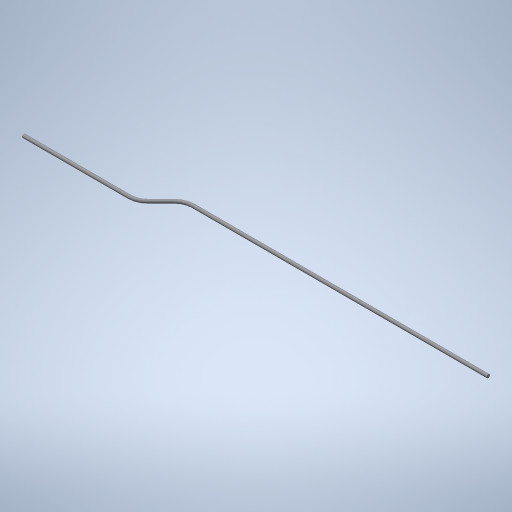
# Autodesk Inventor part: cable medio
Saved by Autodesk Inventor 2023 (Build 270158000, 158)
## iProperties
Created: 2022-10-18
Part Number: cable medio
Material: Generic
Document SubType Name: Modeling
Designer: Xiaba
Density: 1 g/cm^3
Appearance: Default
Author: Xiaba
Autodesk Inventor part; units mm, degrees
ref_plane "YZ Plane" through (0, 0, 0) normal (1, 0, 0) x (0, 1, 0)
ref_plane "XZ Plane" through (0, 0, 0) normal (0, 1, 0) x (-1, 0, 0)
ref_plane "XY Plane" through (0, 0, 0) normal (0, 0, 1) x (1, 0, 0)
sketch "Sketch1" plane through (0, 0, 0) normal (1, 0, 0) x (0, 1, 0)
  circle A0 centre (0, 0) radius 0.45
  dimension "d0" = 0.9
  constraints: 1 centre point, 1 coincident
  measures "d0" diameter of A0
sketch "Sketch2" plane through (0, 0, 0) normal (0, 1, 0) x (-1, 0, 0)
  line L0 (0, 0) -> (0.1, 0)
  line L1 (0.1, 0) -> (78.0289, 0)
  line L2 (81.5645, 1.4645) -> (84.9995, 4.8995)
  line L3 (88.535, 6.364) -> (116.464, 6.364)
  arc A0 (88.535, 6.364) -> (84.9995, 4.8995) centre (88.535, 1.364) ccw
  arc A1 (78.0289, 0) -> (81.5645, 1.4645) centre (78.0289, 5) ccw
  point P0 (80.1, 0)
  point P1 (86.464, 6.364)
  dimension "d1" = 0.1
  dimension "d4" = 80
  dimension "d6" = 9
  dimension "d7" = 30
  dimension "d8" = 5
  constraints: 8 end point, 4 point on circle, 4 point on line, 4 tangent, 3 horizontal, 2 centre point, 1 equal radius
  measures "d1" distance of L0.start L0.end
  measures "d4" distance of L0.end point (80.1, 0)
  measures "d6" distance of point (80.1, 0) point (86.464, 6.364)
  measures "d7" distance of point (86.464, 6.364) L3.end
  measures "d8" radius of A0
sweep "Sweep2" add profiles "Sketch1" path "Sketch2"
body "Solid2"
